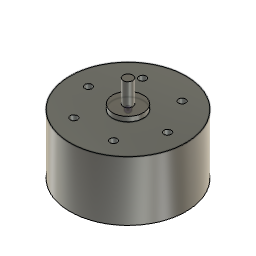
dc_motor_model (Autodesk Fusion 360 design; units mm, degrees)
Autodesk Fusion 360 part; units mm, degrees
sketch "Sketch1" plane through (0, 0, 0) normal (0, 0, 1) x (1, 0, 0)
  circle A0 centre (0, 0) radius 12.07
  circle A1 centre (0, 0) radius 3.2
  dimension "d1" = 24.14
  dimension "d2" = 6.4
  constraint coincident A0.centre A1.centre
  constraint concentric A0 A1
  measures "d1" diameter of A0
  measures "d2" diameter of A1
extrude "Extrude1" add sketch "Sketch1" against normal blind 12.4 contours A0 | A1
extrude "Extrude2" add sketch "Sketch1" along normal blind 1 contours A1
sketch "Sketch2" plane through (0, 0, 1) normal (0, 0, 1) x (-1, 0, 0)
  circle A0 centre (0, 0) radius 3.2
  circle A1 centre (0, 0) radius 1
  dimension "d7" = 2
  constraint coincident A0.centre A1.centre
  measures "d7" diameter of A1
extrude "Extrude3" add sketch "Sketch2" along normal blind 4.7 contours A1
sketch "Sketch3" plane through (0, 0, 0) normal (0, 0, 1) x (1, 0, 0)
  line L0 (0, 0) -> (-8.25, 0) construction
  circle A0 centre (-8.25, 0) radius 0.75
  circle A1 centre (-4.125, -7.1447) radius 0.75
  circle A2 centre (4.125, -7.1447) radius 0.75
  circle A3 centre (8.25, 0) radius 0.75
  circle A4 centre (4.125, 7.1447) radius 0.75
  circle A5 centre (-4.125, 7.1447) radius 0.75
  dimension "d10" = 8.25
  dimension "d11" = 1.5
  dimension "d13" = 360
  constraint coincident L0.start origin
  constraint horizontal L0
  constraint coincident L0.end A0.centre
  measures "d10" distance of L0.start L0.end
  measures "d11" diameter of A0
extrude "Extrude4" cut sketch "Sketch3" against normal blind 2
